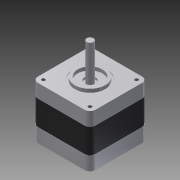
# Autodesk Inventor part: nema17 38mm
Saved by Autodesk Inventor 2013 (Build 170138000, 138)
## iProperties
Created: 2014-01-18
Part Number: nema17 38mm
Material: Generic
Document SubType Name: Modeling
Designer: Masta
Density: 1 g/cm^3
Author: Masta
Autodesk Inventor part; units mm, degrees
ref_plane "YZ Plane" through (0, 0, 0) normal (1, 0, 0) x (0, 1, 0)
sketch "Sketch1" plane through (0, 0, 0) normal (0, 0, 1) x (1, 0, 0)
  circle A0 centre (0, 0) radius 12.5
  circle A1 centre (0, 0) radius 9
  circle A2 centre (0, 0) radius 11
  line L0 (17, -21) -> (-17, -21)
  line L1 (-21, -17) -> (-21, 17)
  line L2 (-17, 21) -> (17, 21)
  line L3 (21, 17) -> (21, -17)
  line L4 (21, -21) -> (-21, 21) construction
  line L5 (-21, -21) -> (21, 21) construction
  arc A3 (-17, 21) -> (-21, 17) centre (-17, 17) ccw
  arc A4 (-21, -17) -> (-17, -21) centre (-17, -17) ccw
  arc A5 (17, -21) -> (21, -17) centre (17, -17) ccw
  arc A6 (21, 17) -> (17, 21) centre (17, 17) ccw
  line L6 (15.5, -15.5) -> (-15.5, -15.5) construction
  line L7 (-15.5, -15.5) -> (-15.5, 15.5) construction
  line L8 (-15.5, 15.5) -> (15.5, 15.5) construction
  line L9 (15.5, 15.5) -> (15.5, -15.5) construction
  line L10 (15.5, -15.5) -> (-15.5, 15.5) construction
  line L11 (-15.5, -15.5) -> (15.5, 15.5) construction
  circle A7 centre (0, 0) radius 2.5
  circle A8 centre (0, 0) radius 4
  dimension "d0" = 42
  dimension "d2" = 42
  dimension "d3" = 4
  dimension "d4" = 18
  dimension "d5" = 22
  dimension "d6" = 25
  dimension "d7" = 31
  dimension "d22" = 5
  dimension "d23" = 8
  constraints: 24 end point, 10 point on line, 9 centre point, 8 coincident, 8 point on circle, 8 tangent, 4 midpoint, 4 parallel, 3 equal radius, 2 horizontal, 2 perpendicular
  measures "d0" distance of L4.end L5.end
  measures "d2" distance of L5.start L4.end
  measures "d3" radius of A3
  measures "d4" diameter of A1
  measures "d5" diameter of A2
  measures "d6" diameter of A0
  measures "d7" distance of L7.end L8.end
  measures "d22" diameter of A7
  measures "d23" diameter of A8
ref_plane "Work Plane1" through (0, 0, -10) normal (0, 0, 1) x (1, 0, 0)
ref_plane "Work Plane3" through (0, 0, -28) normal (0, 0, 1) x (1, 0, 0)
ref_plane "Work Plane2" through (0, 0, -38) normal (0, 0, 1) x (1, 0, 0)
extrude "Extrusion1" add sketch "Sketch1" against normal up to surface (10 mm away) from surface at 0 contours A0 | A1 | A2 | L0 A4 L1 A3 L2 A6 L3 A5 | A7 | A8
sketch "Sketch2" plane through (17, 21, -10) normal (0, 0, -1) x (-1, 0, 0)
  arc A0 (34, -42) -> (38, -38) centre (34, -38) ccw projected
  line L0 (38, -38) -> (38, -4) projected
  arc A1 (38, -4) -> (34, 0) centre (34, -4) ccw projected
  line L1 (34, 0) -> (0, 0) projected
  arc A2 (0, 0) -> (-4, -4) centre (0, -4) ccw projected
  line L2 (-4, -4) -> (-4, -38) projected
  arc A3 (-4, -38) -> (0, -42) centre (0, -38) ccw projected
  line L3 (0, -42) -> (34, -42) projected
  line L4 (0, -0.1) -> (34, -0.1)
  arc A4 (37.9, -4) -> (34, -0.1) centre (34, -4) ccw
  line L5 (37.9, -4) -> (37.9, -38)
  arc A5 (34, -41.9) -> (37.9, -38) centre (34, -38) ccw
  line L6 (34, -41.9) -> (0, -41.9)
  arc A6 (-3.9, -38) -> (0, -41.9) centre (0, -38) ccw
  line L7 (-3.9, -38) -> (-3.9, -4)
  arc A7 (0, -0.1) -> (-3.9, -4) centre (0, -4) ccw
  point P0 (17, -21)
  dimension "d13" = 0.1
  constraints: 8 end point, 8 point on circle, 4 centre point, 7 other
  measures "d13" distance between parallel lines of L1 L4
extrude "Extrusion2" add sketch "Sketch2" along normal up to surface (10 mm away) from surface at 18 contours L3 A3 L2 A2 L1 A1 L0 A0 | L4 A4 L5 A5 L6 A6 L7 A7
extrude "Extrusion3" add sketch "Sketch2" along normal up to surface (18 mm away) from surface at 0 contours L4 A4 L5 A5 L6 A6 L7 A7
extrude "Extrusion4" cut sketch "Sketch1" against normal blind 0.5 contours A0 | A1 | A8
extrude "Extrusion5" add sketch "Sketch1" along normal blind 2 contours A2
extrude "Extrusion6" cut sketch "Sketch1" against normal blind 2 contours A8
extrude "Extrusion7" add sketch "Sketch1" along normal blind 25 contours A7
hole "Hole1" at (-17, 17, 0) at (-17, -17, 0) at (17, -17, 0) at (17, 17, 0) direction (0, 0, -1) diameter 2.459 depth 4 tip angle 118 thread size "M3x0.5" class "6H" standard "ISO Metric profile"
body "Solid1"
